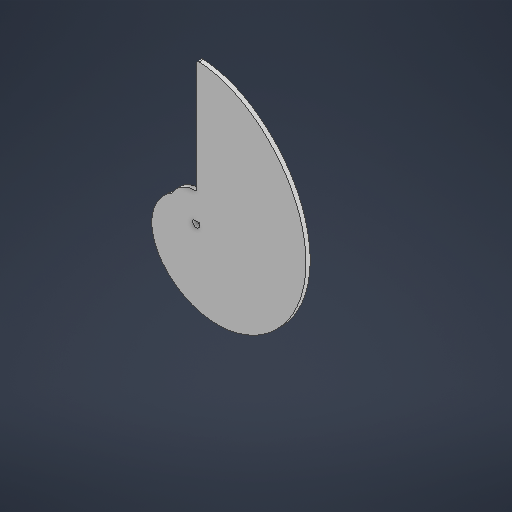
# Autodesk Inventor part: Cam_arche1
Saved by Autodesk Inventor 2027 (Build 310192000, 192)
## iProperties
Created: 2026-05-25
Part Number: Cam_arche1
Material: Generic
Document SubType Name: Modeling
Designer: alexy
Density: 1 g/cm^3
Appearance: Default
Author: alexy
Autodesk Inventor part; units mm, degrees
ref_plane "YZ Plane" through (0, 0, 0) normal (1, 0, 0) x (0, 1, 0)
ref_plane "XZ Plane" through (0, 0, 0) normal (0, 1, 0) x (-1, 0, 0)
ref_plane "XY Plane" through (0, 0, 0) normal (0, 0, 1) x (1, 0, 0)
sketch "Sketch1" plane through (0, 0, 0) normal (0, 0, 1) x (1, 0, 0)
  circle A0 centre (0, 0) radius 100
  circle A1 centre (0, 0) radius 20
  arc A2 (72.7461, -42) -> (0, 84) centre (0, 0) ccw
  arc A3 (0, -68) -> (0, 68) centre (0, 0) ccw
  arc A4 (-31.1769, 18) -> (31.1769, 18) centre (0, 0) ccw
  arc A5 (-45.0333, -26) -> (45.0333, 26) centre (0, 0) ccw
  line L0 (0, 0) -> (0, 100)
  line L1 (0, 0) -> (-86.6025, 50)
  line L2 (0, 0) -> (-86.6025, -50)
  line L3 (0, 0) -> (0, -100)
  line L4 (0, 0) -> (86.6025, -50)
  line L5 (0, 0) -> (86.6025, 50)
  spline S0 degree 3 poles (0, 84) (73.4224, 56.463) (45.742, -47.7639) (0, -20) knots 0 0 0 0 1 1 1 1
  circle A6 centre (0, 0) radius 10
  spline S1 degree 4 poles (0, 100) (55.6412, 98.6208) (125.3971, 4.9821) (11.8678, -111.8252) (-57.9765, -4.8676) (-8.1188, 21.3354) (0, 10) knots 0 0 0 0 0 0.510428 0.679825 1 1 1 1 1
  point P0 (31.1769, -18)
  point P1 (17.3205, 10)
  point P2 (8.6603, 5)
  point P3 (17.3205, 10)
  point P4 (72.7461, 42)
  point P5 (58.8897, -34)
  point P6 (0, -52)
  point P7 (-31.1769, -18)
  point P8 (-17.3205, 10)
  point P9 (0, 20)
  dimension "d0" = 200
  dimension "d24" = 20
  dimension "d1" = 40
  dimension "d2" = 168
  dimension "d3" = 136
  dimension "d4" = 104
  dimension "d5" = 72
  dimension "d9" = 360
  constraints: 17 point on line, 16 point on circle, 12 end point, 8 coincident, 5 centre point, 1 vertical, 36 other
  measures "d1" diameter of A1
  measures "d2" diameter of A2
  measures "d3" diameter of A3
  measures "d4" diameter of A5
  measures "d5" diameter of A4
extrude "Extrusion1" add sketch "Sketch1" along normal blind 3 contours S1 A2 L0 | L5 A3 S0 A2 | S1 A3 L5 | S0 A3 L0 | L5 S0 A3 | A3 L4 A5 L5 | S1 A5 L4 | A3 S0 L5 A1 L0 | S0 A4 L5 | A5 L4 S0 | A5 L3 A4 L4 | S1 A4 L3 | L2 A1 L3 A4 | S1 A1 L2 | L1 A6 L2 A1 | S1 A6 L1 | A1 L0 S1 | A1 L5 A6 L0 | A4 L4 A1 L5 | S0 A1 L4 | A4 L3 S0 | L2 A6 L3 A1 | A6 L0 L1 | L1 L2 A6 | A6 L5 L0 | A1 L4 A6 L5 | A1 L3 A6 L4 | L2 L3 A6 | L4 A6 L3 | L5 A6 L4
fillet "Fillet1" radius 2 1 edges at (0, 100, 1.5)
sketch "Sketch3" plane through (0, 0, 3) normal (0, 0, 1) x (1, 0, 0)
  circle A0 centre (0, 0) radius 2.5
  line L0 (-2.0712, 1.4) -> (2.0712, 1.4)
  dimension "d19" = 5
  dimension "d20" = 1.4
  constraints: 2 end point, 2 point on circle, 1 centre point, 1 coincident, 1 horizontal
  measures "d19" diameter of A0
  measures "d20" distance from line of point (0, 0) L0
extrude "Extrusion3" cut sketch "Sketch3" against normal blind 3 contours A0 L0 picked at (0.0636, 0.1024)
equation "\"d2\" = 0.8 * d0 + 0.2 * d1"
equation "\"d3\" = 0.6 * d0 + 0.4 * d1"
equation "\"d4\" = 0.4 * d0 + 0.6 * d1"
equation "\"d5\" = 0.2 * d0 + 0.8 * d1"
body "Solid1"
